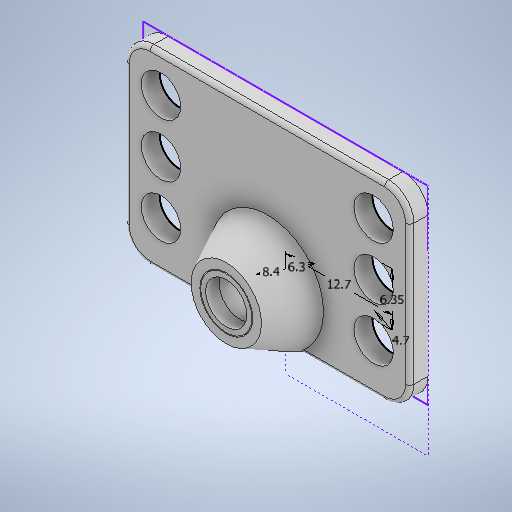
# Autodesk Inventor part: RevMagnetHolder-1inchmounts
Saved by Autodesk Inventor 2025 (Build 290162000, 162)
## iProperties
Created: 2025-02-22
Part Number: RevMagnetHolder-1inchmounts
Material: Generic
Document SubType Name: Modeling
Designer: john
Density: 1 g/cm^3
Appearance: Default
Author: john
Autodesk Inventor part; units mm, degrees
ref_plane "YZ Plane" through (0, 0, 0) normal (1, 0, 0) x (0, 1, 0)
ref_plane "XZ Plane" through (0, 0, 0) normal (0, 1, 0) x (-1, 0, 0)
ref_plane "XY Plane" through (0, 0, 0) normal (0, 0, 1) x (1, 0, 0)
sketch "Sketch1" plane through (0, 0, 0) normal (0, 0, 1) x (1, 0, 0)
  circle A0 centre (0, 0) radius 3.15
  line L0 (0, 0) -> (12.7, 0) construction
  circle A1 centre (12.7, 0) radius 2.35
  line L1 (0, 0) -> (0, 14.467027) construction
  circle A2 centre (12.7, 6.35) radius 2.35
  circle A3 centre (12.7, 12.7) radius 2.35
  line L2 (0, -10.866161) -> (0, 17.080603) construction
  line L3 (0, 17.080603) -> (17.008013, 17.080603) construction
  line L4 (17.008013, 17.080603) -> (17.008013, -10.866161) construction
  line L5 (17.008013, -10.866161) -> (0, -10.866161) construction
  line L6 (0, 17.080603) -> (17.008013, 17.080603)
  line L7 (17.008013, 17.080603) -> (17.008013, -5.592949)
  line L8 (17.008013, -5.592949) -> (0, -5.592949)
  line L9 (0, -5.592949) -> (0, 17.080603)
  line L10 (0, 17.080603) -> (-17.008013, 17.080603) construction
  line L11 (0, 17.080603) -> (-17.008013, 17.080603)
  line L12 (-17.008013, -5.592949) -> (0, -5.592949)
  circle A4 centre (-12.7, 0) radius 2.35
  circle A5 centre (-12.7, 6.35) radius 2.35
  circle A6 centre (-12.7, 12.7) radius 2.35
  line L13 (-17.008013, 17.080603) -> (-17.008013, -5.592949)
  circle A7 centre (0, 0) radius 5.592949
  circle A8 centre (0, 0) radius 4.2
  dimension "d0" = 6.3
  dimension "d1" = 12.7
  dimension "d2" = 4.7
  dimension "d5" = 6.35
  dimension "d12" = 8.4
  constraints: 28 end point, 8 centre point, 5 coincident, 5 equal length, 5 symmetric about line, 3 vertical, 2 perpendicular, 1 horizontal, 1 vertical alignment, 9 other
  measures "d0" diameter of A0
  measures "d1" distance of L0.start L0.end
  measures "d2" diameter of A1
  measures "d5" distance of A1.centre A2.centre
  measures "d12" diameter of A8
sketch "Sketch1 outline for Extrusion1" plane through (0, 0, 0) normal (0, 0, 1) x (1, 0, 0)
  line L0 (0, 17.080603) -> (-17.008013, 17.080603)
  line L1 (17.008013, 17.080603) -> (0, 17.080603)
  line L2 (-17.008013, 17.080603) -> (-17.008013, -5.592949)
  line L3 (17.008013, -5.592949) -> (17.008013, 17.080603)
  line L4 (-17.008013, -5.592949) -> (0, -5.592949)
  line L5 (0, -5.592949) -> (17.008013, -5.592949)
  circle A0 centre (-12.7, 0) radius 2.35
  circle A1 centre (0, 0) radius 3.15
  circle A2 centre (12.7, 0) radius 2.35
  circle A3 centre (-12.7, 6.35) radius 2.35
  circle A4 centre (-12.7, 12.7) radius 2.35
  circle A5 centre (12.7, 6.35) radius 2.35
  circle A6 centre (12.7, 12.7) radius 2.35
extrude "Extrusion1" add sketch "Sketch1 outline for Extrusion1" along normal blind 2.2
sketch "Sketch1 outline for Extrusion3" plane through (0, 0, 0) normal (0, 0, 1) x (1, 0, 0)
  circle A0 centre (0, 0) radius 4.2
  circle A1 centre (0, 0) radius 3.15
extrude "Extrusion3" add sketch "Sketch1 outline for Extrusion3" along normal blind 7.1
chamfer "Chamfer1" distance 2.5 distance2 4.9 1 edges at (-4.2, 0, 2.2)
sketch "Sketch2" plane through (0, 0, 7.1) normal (0, 0, 1) x (1, 0, 0)
  circle A0 centre (0, 0) radius 2.45
  circle A1 centre (0, 0) radius 3.05
  dimension "d20" = 4.9
  constraints: 2 centre point, 2 coincident
  measures "d20" diameter of A0
sketch "Sketch2 outline for Extrusion4" plane through (0, 0, 7.1) normal (0, 0, 1) x (1, 0, 0)
  circle A0 centre (0, 0) radius 3.05
  circle A1 centre (0, 0) radius 2.45
extrude "Extrusion4" add sketch "Sketch2 outline for Extrusion4" against normal blind 1.6
fillet "Fillet1" radius 3 4 edges at (-17.008, -5.5929, 1.1) (17.008, -5.5929, 1.1) (17.008, 17.0806, 1.1) (-17.008, 17.0806, 1.1)
fillet "Fillet2" radius 0.5 8 edges at (-16.1293, 16.2019, 2.2) (-17.008, 5.7438, 2.2) (-16.1293, -4.7143, 2.2) (8.8485, -5.5929, 2.2) (16.1293, 16.2019, 2.2) (17.008, 5.7438, 2.2) (16.1293, -4.7143, 2.2) (0, 17.0806, 2.2)
body "Solid1"
